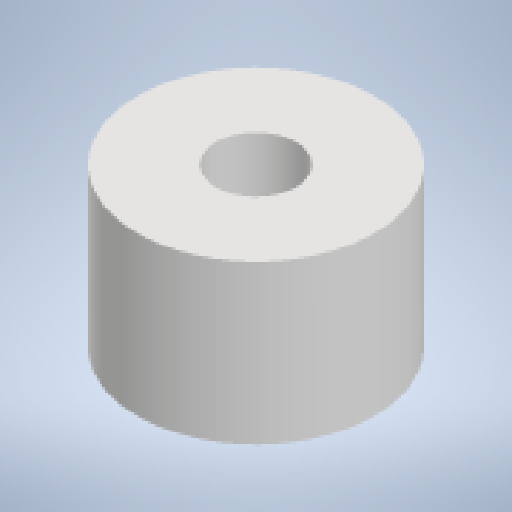
# Autodesk Inventor part: Ballbearing
Saved by Autodesk Inventor 2023 (Build 270158000, 158)
## iProperties
Created: 2023-02-18
Part Number: Ballbearing
Material: Iron, Gray
Document SubType Name: Modeling
Designer: phill
Density: 7.15 g/cm^3
Appearance: Iron Gray
Author: phill
Autodesk Inventor part; units mm, degrees
ref_plane "YZ Plane" through (0, 0, 0) normal (1, 0, 0) x (0, 1, 0)
ref_plane "XZ Plane" through (0, 0, 0) normal (0, 1, 0) x (-1, 0, 0)
sketch "Sketch1" plane through (0, 0, 0) normal (0, 1, 0) x (-1, 0, 0)
  circle A0 centre (0, -107) radius 0.5 projected
  circle A1 centre (0, -107) radius 1.5 projected
  arc A2 (5.6174, 110) -> (3.5, -110) centre (11433.5, -110) ccw projected
  line L0 (3.5, -110) -> (-3.5, -110) projected
  arc A3 (-3.5, -110) -> (-5.6174, 110) centre (-11433.5, -110) ccw projected
  line L1 (-5.6174, 110) -> (5.6174, 110) projected
  point P0 (0, 0)
ref_plane "Work Plane1" through (-0.5, -2, -107.5) normal (0, -1, 0) x (1, 0, 0)
extrude "Extrusion1" add sketch "Sketch1" against normal up to surface (2 mm away) contours A1
body "Solid1"
